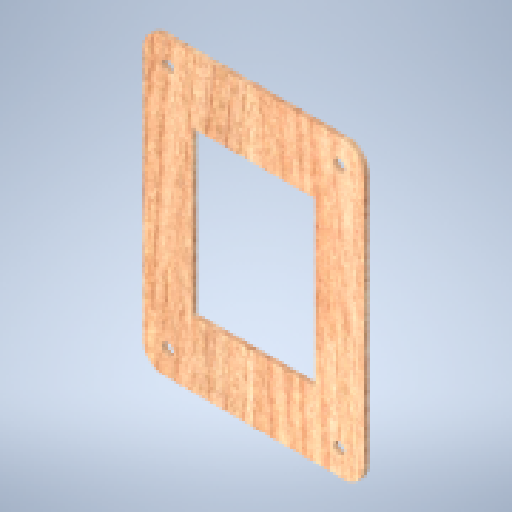
# Autodesk Inventor part: TapaBC
Saved by Autodesk Inventor 2023.1 (Build 271208000, 208)
## iProperties
Created: 2022-11-11
Part Number: TapaBC
Material: MDF Medium Density Fiberboard
Document SubType Name: Modeling
Designer: Daniel Peña
Density: 0.8 g/cm^3
Appearance: Birch - Natural Polished
Author: Daniel Peña
Autodesk Inventor part; units mm, degrees
ref_plane "YZ Plane" through (0, 0, 0) normal (1, 0, 0) x (0, 1, 0)
ref_plane "XZ Plane" through (0, 0, 0) normal (0, 1, 0) x (-1, 0, 0)
ref_plane "XY Plane" through (0, 0, 0) normal (0, 0, 1) x (1, 0, 0)
sketch "Sketch1" plane through (0, 0, 0) normal (0, 0, 1) x (1, 0, 0)
  line L0 (-71.2144, 83.3219) -> (39.7856, 83.3219)
  line L1 (51.7856, 71.3219) -> (51.7856, -84.6781)
  line L2 (39.7856, -96.6781) -> (-71.2144, -96.6781)
  line L3 (-83.2144, -84.6781) -> (-83.2144, 71.3219)
  line L4 (-53.2144, 43.3219) -> (21.7856, 43.3219)
  line L5 (21.7856, 43.3219) -> (21.7856, -56.6781)
  line L6 (21.7856, -56.6781) -> (-53.2144, -56.6781)
  line L7 (-53.2144, -56.6781) -> (-53.2144, 43.3219)
  arc A0 (-71.2144, 83.3219) -> (-83.2144, 71.3219) centre (-71.2144, 71.3219) ccw
  arc A1 (51.7856, 71.3219) -> (39.7856, 83.3219) centre (39.7856, 71.3219) ccw
  arc A2 (39.7856, -96.6781) -> (51.7856, -84.6781) centre (39.7856, -84.6781) ccw
  arc A3 (-83.2144, -84.6781) -> (-71.2144, -96.6781) centre (-71.2144, -84.6781) ccw
  point P0 (0, 0)
  point P1 (-83.2144, 83.3219)
  point P2 (51.7856, -96.6781)
  point P3 (51.7856, 83.3219)
  point P4 (-83.2144, -96.6781)
  dimension "d0" = 180
  dimension "d2" = 100
  dimension "d3" = 40
  dimension "d4" = 40
  dimension "d7" = 30
  dimension "d8" = 30
  dimension "d10" = 75
  dimension "d11" = 12
  constraints: 16 end point, 8 point on circle, 8 point on line, 8 tangent, 4 centre point, 4 parallel, 3 equal radius, 2 horizontal, 2 perpendicular
  measures "d0" distance of point (-83.214, -96.678) point (-83.214, 83.322)
  measures "d2" distance between parallel lines of L6 L4
  measures "d3" distance between parallel lines of L0 L4
  measures "d4" distance between parallel lines of L2 L6
  measures "d7" distance between parallel lines of L7 L3
  measures "d8" distance between parallel lines of L1 L5
  measures "d10" distance between parallel lines of L5 L7
  measures "d11" radius of A0
extrude "Extrusion1" add sketch "Sketch1" along normal blind 3
sketch "Sketch3" plane through (0, 0, 3) normal (0, 0, 1) x (1, 0, 0)
  line L0 (39.7856, 83.3219) -> (-71.2144, 83.3219) construction
  line L1 (-15.7144, 83.3219) -> (-15.7144, -96.6781) construction
  line L2 (-71.2144, -96.6781) -> (39.7856, -96.6781) construction
  line L3 (-83.2144, 71.3219) -> (-83.2144, -84.6781) construction
  line L4 (-83.2144, -6.6781) -> (51.7856, -6.6781) construction
  line L5 (51.7856, -84.6781) -> (51.7856, 71.3219) construction
  point P0 (0, 0)
  point P1 (-68.2144, 68.3219)
  point P2 (36.7856, 68.3219)
  point P3 (36.7856, -81.6781)
  point P4 (-68.2144, -81.6781)
  dimension "d12" = 15
  dimension "d13" = 15
  constraints: 4 end point, 4 midpoint, 3 symmetric about line
  measures "d12" distance from line of L3 point (-68.214, 68.322)
  measures "d13" distance from line of point (-68.214, 68.322) L0
hole "Hole1" at (-68.2144, 68.3219, 3) at (36.7856, 68.3219, 3) at (36.7856, -81.6781, 3) at (-68.2144, -81.6781, 3) direction (0, 0, -1) diameter 7 end through all
equation "\"d3\" = d4"
equation "\"d8\" = d7"
body "Solid1"
